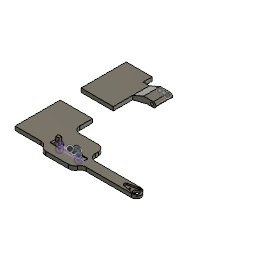
Arm (Autodesk Fusion 360 design; units mm, degrees)
part number: 2026-03-16-20-26-23-192
Autodesk Fusion 360 part; units mm, degrees
sketch "Sketch1" plane through (0, 0, 0) normal (0, 0, 1) x (1, 0, 0)
  circle A0 centre (0, 0) radius 2.9
  circle A1 centre (0, 0) radius 7.5
  line L0 (0, 0) -> (0, 7.5)
  line L1 (0, 0) -> (0, -7.5)
  line L2 (0, 7.5) -> (-100, 7.5)
  line L3 (0, -7.5) -> (-71, -7.5)
  line L4 (-100, -32.5) -> (-100, 7.5)
  line L5 (-100, 7.5) -> (-180, 7.5)
  line L6 (-180, 7.5) -> (-180, -32.5)
  line L7 (-120, -32.5) -> (-100, -32.5)
  line L8 (-100, -32.5) -> (-100, -26.5)
  line L9 (-180, 7.5) -> (-130, 7.5)
  line L10 (-130, -42.5) -> (-130, -62.5)
  line L11 (-130, -62.5) -> (-180, -62.5)
  line L12 (-180, -62.5) -> (-180, 7.5)
  arc A2 (-120, -32.5) -> (-130, -42.5) centre (-120, -42.5) ccw
  line L13 (-81, -7.5) -> (-100, -7.5)
  line L14 (-100, -7.5) -> (-100, -32.5)
  line L15 (-100, -32.5) -> (-91, -32.5)
  line L16 (-81, -22.5) -> (-81, -17.5)
  arc A3 (-71, -7.5) -> (-81, -17.5) centre (-71, -17.5) ccw
  arc A4 (-91, -32.5) -> (-81, -22.5) centre (-91, -22.5) ccw
  line L17 (-79.7998, 7.5) -> (-129.7998, 7.5)
  line L18 (-129.7998, 7.5) -> (-129.7998, 17.5)
  line L19 (-129.7998, 17.5) -> (-79.7998, 17.5)
  line L20 (-79.7998, 17.5) -> (-79.7998, 7.5)
  point P0 (-100, -7.5)
  dimension "d3" = 5.8
  dimension "d5" = 15
  dimension "d6" = 7.5
  dimension "d7" = 7.5
  dimension "d10" = 100
  dimension "d11" = 100
  dimension "d13" = 40
  dimension "d14" = 80
  dimension "d15" = 40
  dimension "d16" = 50
  dimension "d17" = 70
  dimension "d19" = 10
  dimension "d52" = 10
  dimension "d71" = 50
  dimension "d72" = 10
  constraint coincident A0.centre A1.centre
  constraint concentric A0 A1
  constraint vertical L0
  constraint parallel L0 L1
  constraint perpendicular L0 L2
  constraint perpendicular L1 L3
  constraint vertical L4
  constraint horizontal L5
  constraint vertical L6
  constraint horizontal L7
  constraint vertical L8
  constraint horizontal L9
  constraint vertical L10
  constraint horizontal L11
  constraint vertical L12
  constraint coincident L2.end L8
  constraint coincident P0 L3
  constraint coincident L6.end L7
  constraint coincident L9.end L10
  constraint tangent L7 A2
  constraint tangent L10 A2
  constraint horizontal L13
  constraint vertical L14
  constraint horizontal L15
  constraint vertical L16
  constraint coincident L13.start L16
  constraint coincident L3 L13.start
  constraint tangent L16 A3
  constraint tangent L3 A3
  constraint tangent L15 A4
  constraint tangent L16 A4
  constraint equal A3 A4
  constraint horizontal L17
  constraint vertical L18
  constraint horizontal L19
  constraint vertical L20
  constraint coincident L2 L17.start
  measures "d3" diameter of A0
  measures "d5" diameter of A1
  measures "d6" distance of A0.centre L0.end
  measures "d7" distance of A0.centre L1.end
  measures "d10" distance of L0.end L2.end
  measures "d11" distance of L1.end P0
  measures "d13" distance of L2.end L4.start
  measures "d14" distance of L2.end L5.end
  measures "d15" distance of L2.end L4.start
  measures "d16" distance of L5.end L9.end
  measures "d17" distance of L5.end L11.end
  measures "d19" radius of A2
  measures "d52" radius of A3
  measures "d71" distance of L17.start L17.end
  measures "d72" distance of L17.start L19.end
extrude "Extrude1" add sketch "Sketch1" along normal blind 6 contours A0 A1 L0 L1 | A0 A1 L0 L1 | A1 L2 L3 L4 L8 L14 L15 L16 A3 A4 L17 | L2 L5 L17 L18 L19 L20 | L4 L5 L6 L7 L8 L9 L10 L11 L12 A2 L14 L17 makes body 1
move_body "Move1" bodies 1 to x (1, 0, 0) y (0, 0, 1) z (0, -1, 0) at (0, -14.492, 14.492)
move_body "Move2" bodies 1 to x (1, 0, 0) y (0, 1, 0) z (0, 0, 1) at (0, 21, 0)
sketch "Sketch2" plane through (0, 6.508, 0) normal (0, 1, 0) x (-1, 0, 0)
  line L0 (91, -18.008) -> (120, -18.008)
  arc A0 (130, -28.008) -> (120, -18.008) centre (120, -28.008) ccw
  line L1 (130, -28.008) -> (130, -48.008)
  line L2 (130, -48.008) -> (180, -48.008)
  line L3 (180, -48.008) -> (180, 21.992)
  line L4 (180, 21.992) -> (129.7998, 21.992)
  arc A1 (0, 21.992) -> (0, 6.992) centre (0, 14.492) ccw
  line L5 (0, 6.992) -> (71, 6.992)
  line L6 (89, 17) -> (94, 17)
  line L7 (94, 17) -> (94, 13)
  line L8 (94, 13) -> (89, 13)
  line L9 (89, 13) -> (89, 17)
  arc A2 (81, -3.008) -> (71, 6.992) centre (71, -3.008) ccw
  line L10 (81, -3.008) -> (81, -8.008)
  arc A3 (81, -8.008) -> (91, -18.008) centre (91, -8.008) ccw
  line L11 (129.7998, 21.992) -> (129.7998, 31.992)
  line L12 (129.7998, 31.992) -> (79.7998, 31.992)
  line L13 (79.7998, 31.992) -> (79.7998, 21.992)
  line L14 (79.7998, 21.992) -> (0, 21.992)
  circle A4 centre (0, 14.492) radius 2.9
  dimension "d22" = 5
  dimension "d23" = 4
  constraint horizontal L6
  constraint vertical L7
  constraint horizontal L8
  constraint vertical L9
  measures "d22" distance of L6.start L6.end
  measures "d23" distance of L6.start L8.end
extrude "Extrude2" add sketch "Sketch2" along normal blind 13 contours L6 L7 L8 L9 bodies 1
sketch "Sketch3" plane through (0, 0, 13) normal (0, 0, -1) x (-1, 0, 0)
  line L0 (94, 6.508) -> (94, 19.508)
  line L1 (94, 19.508) -> (89, 19.508)
  line L2 (89, 19.508) -> (89, 6.508)
  line L3 (92.4, 13.058) -> (91.45, 13.058)
  circle A0 centre (91.45, 13.058) radius 0.95
  line L4 (120, 6.508) -> (91, 6.508)
  line L5 (91, 0.508) -> (120, 0.508)
  line L6 (120, 0.508) -> (120, 6.508)
  line L7 (91.45, 13.058) -> (91.45, 6.508)
  line L8 (91.45, 13.058) -> (94, 13.058)
  line L9 (91, 6.508) -> (91, 0.508)
  line L10 (89, 6.508) -> (94, 6.508)
  dimension "d33" = 0.95
  constraint coincident L3.end A0.centre
  constraint coincident L3.start A0
  constraint coincident L4 L7.end
  constraint perpendicular L4 L7
  constraint coincident L0 L8.end
  constraint perpendicular L0 L8
  measures "d33" distance of L3.start L3.end
extrude "Extrude3" cut sketch "Sketch3" against normal blind 10 contours L3 A0 L7 L8 | L3 A0 L7 L8 bodies 1
sketch "Sketch4" plane through (0, 6.508, 0) normal (0, 1, 0) x (-1, 0, 0)
  line L0 (94, 17) -> (94, 13)
  line L1 (91, -18.008) -> (120, -18.008)
  arc A0 (130, -28.008) -> (120, -18.008) centre (120, -28.008) ccw
  line L2 (130, -28.008) -> (130, -48.008)
  line L3 (130, -48.008) -> (180, -48.008)
  line L4 (180, -48.008) -> (180, 21.992)
  line L5 (180, 21.992) -> (129.7998, 21.992)
  arc A1 (0, 21.992) -> (0, 6.992) centre (0, 14.492) ccw
  line L6 (0, 6.992) -> (71, 6.992)
  line L7 (94, 17) -> (116.7, 17)
  arc A2 (81, -3.008) -> (71, 6.992) centre (71, -3.008) ccw
  line L8 (81, -3.008) -> (81, -8.008)
  arc A3 (81, -8.008) -> (91, -18.008) centre (91, -8.008) ccw
  line L9 (116.7, 17) -> (116.8, 17)
  line L10 (116.8, 17) -> (121.8, 17)
  line L11 (121.8, 17) -> (121.8, 13)
  line L12 (121.8, 13) -> (116.8, 13)
  line L13 (116.8, 13) -> (116.8, 17)
  line L14 (89, 13) -> (89, 17)
  line L15 (89, 17) -> (94, 17)
  line L16 (94, 13) -> (89, 13)
  line L17 (129.7998, 21.992) -> (129.7998, 31.992)
  line L18 (129.7998, 31.992) -> (79.7998, 31.992)
  line L19 (79.7998, 31.992) -> (79.7998, 21.992)
  line L20 (79.7998, 21.992) -> (0, 21.992)
  circle A4 centre (0, 14.492) radius 2.9
  dimension "d38" = 22.7
  dimension "d53" = 0.1
  dimension "d54" = 5
  dimension "d55" = 4
  constraint coincident L0 L7.start
  constraint perpendicular L0 L7
  constraint horizontal L9
  constraint horizontal L10
  constraint vertical L11
  constraint horizontal L12
  constraint vertical L13
  measures "d38" distance of L0.start L7.end
  measures "d53" distance of L7.end L9.end
  measures "d54" distance of L9.end L10.end
  measures "d55" distance of L9.end L12.end
extrude "Extrude4" add sketch "Sketch4" along normal blind 13 contours L10 L11 L12 L13 bodies 1
sketch "Sketch6" plane through (0, 0, 13) normal (0, 0, -1) x (-1, 0, 0)
  line L0 (121.8, 6.508) -> (121.8, 19.508)
  line L1 (121.8, 19.508) -> (116.8, 19.508)
  line L2 (116.8, 19.508) -> (116.8, 6.508)
  line L3 (122.7377, 11.508) -> (116.8, 11.508)
  line L4 (116.8, 11.508) -> (116.8, 6.508)
  line L5 (116.8, 6.508) -> (130.8, 6.508)
  spline S0 degree 3 poles (122.7377, 11.508) (123.0614, 10.8558) (123.4874, 10.2087) (124.46, 9.0768) (125.006, 8.5907) (126.304, 7.6534) (127.188, 7.2097) (129.0062, 6.6373) (129.9408, 6.508) (130.8, 6.508) knots 2.617897 2.617897 2.617897 2.617897 2.836337 2.836337 3.054776 3.054776 3.376245 3.376245 3.697714 3.697714 3.697714 3.697714
  line L6 (120, 6.508) -> (130, 6.508)
  line L7 (120, 6.508) -> (120, 0.508)
  line L8 (130, 0.508) -> (120, 0.508)
  line L9 (130, 0.508) -> (130, 6.508)
  line L10 (120, 6.508) -> (91, 6.508)
  line L11 (91, 6.508) -> (91, 0.508)
  line L12 (91, 0.508) -> (120, 0.508)
  line L13 (120, 0.508) -> (120, 6.508)
  line L14 (116.8, 6.508) -> (119.35, 6.508)
  line L15 (119.35, 6.508) -> (119.35, 13.058)
  line L16 (119.35, 13.058) -> (116.8, 13.058)
  line L17 (116.8, 13.058) -> (116.8, 6.508)
  circle A0 centre (119.35, 13.058) radius 0.95
  line L18 (116.8, 6.508) -> (121.8, 6.508)
  dimension "d73" = 2.55
  dimension "d74" = 6.55
  dimension "d75" = 1.9
  constraint horizontal L14
  constraint vertical L15
  constraint horizontal L16
  constraint vertical L17
  constraint coincident L2.end L4.end
  constraint coincident L15.end L16.start
  measures "d73" distance of L2.end L14.end
  measures "d74" distance of L2.end L16.end
  measures "d75" diameter of A0
extrude "Extrude7" cut sketch "Sketch6" against normal blind 10 contours L15 L16 A0 | L15 L16 A0 bodies 1
fillet "Fillet11" radius 10 2 edges at (-129.7998, 3.508, 21.992) (-79.7998, 3.508, 21.992) on bodies 1
fillet "Fillet12" radius 10 2 edges at (-129.7998, 3.508, 31.992) (-79.7998, 3.508, 31.992) on bodies 1
fillet "Fillet13" radius 9 2 edges at (-121.8, 6.508, 15) (-89, 6.508, 15) on bodies 1
sketch "Sketch7" plane through (0, 6.508, 0) normal (0, 1, 0) x (-1, 0, 0)
  line L0 (94, 17) -> (94, 13)
  line L1 (94, 13) -> (80, 13)
  line L2 (80, 13) -> (80, 17)
  line L3 (130.8, 13) -> (116.8, 13)
  line L4 (116.8, 13) -> (116.8, 17)
  line L5 (130.8, 17) -> (130.8, 13)
  arc A0 (87.1203, 31.992) -> (78.4601, 26.992) centre (87.1203, 21.992) ccw
  arc A1 (69.7998, 21.992) -> (78.4601, 26.992) centre (69.7998, 31.992) ccw
  line L6 (69.7998, 21.992) -> (0, 21.992)
  arc A2 (0, 21.992) -> (0, 6.992) centre (0, 14.492) ccw
  line L7 (0, 6.992) -> (71, 6.992)
  arc A3 (81, -3.008) -> (71, 6.992) centre (71, -3.008) ccw
  line L8 (81, -3.008) -> (81, -8.008)
  arc A4 (81, -8.008) -> (91, -18.008) centre (91, -8.008) ccw
  line L9 (91, -18.008) -> (120, -18.008)
  arc A5 (130, -28.008) -> (120, -18.008) centre (120, -28.008) ccw
  line L10 (130, -28.008) -> (130, -48.008)
  line L11 (130, -48.008) -> (180, -48.008)
  line L12 (180, -48.008) -> (180, 21.992)
  line L13 (180, 21.992) -> (139.7998, 21.992)
  arc A6 (131.1396, 26.992) -> (139.7998, 21.992) centre (139.7998, 31.992) ccw
  arc A7 (131.1396, 26.992) -> (122.4793, 31.992) centre (122.4793, 21.992) ccw
  line L14 (122.4793, 31.992) -> (87.1203, 31.992)
  line L15 (94, 13) -> (94, 8)
  line L16 (94, 8) -> (81, 8)
  line L17 (81, 8) -> (81, -3.008)
  line L18 (94, -3.008) -> (94, 8)
  line L19 (81, 8) -> (180, 8)
  line L20 (180, 8) -> (180, -18.008)
  line L21 (120, -18.008) -> (91, -18.008)
  line L22 (81, -8.008) -> (81, 8)
  line L23 (130, -48.008) -> (180, -48.008)
  line L24 (180, -48.008) -> (180, -18.008)
  line L25 (180, -18.008) -> (130, -18.008)
  line L26 (130, -28.008) -> (130, -48.008)
  arc A8 (81, -8.008) -> (91, -18.008) centre (91, -8.008) ccw
  arc A9 (130, -28.008) -> (120, -18.008) centre (120, -28.008) ccw
  line L27 (180, 8) -> (139.7998, 8)
  line L28 (139.7998, 8) -> (139.7998, 21.992)
  line L29 (139.7998, 21.992) -> (180, 21.992)
  line L30 (180, 21.992) -> (180, 8)
  line L31 (130, -28.008) -> (130, 8)
  circle A10 centre (0, 14.492) radius 2.9
  line L32 (80, 17) -> (94, 17)
  line L33 (116.8, 17) -> (130.8, 17)
  dimension "d84" = 5
  constraint coincident L0.end L1.start
  constraint perpendicular L1 L15
  constraint horizontal L16
  constraint vertical L17
  constraint vertical L18
  constraint coincident A3.start L8.start
  constraint horizontal L19
  constraint vertical L20
  constraint horizontal L21
  constraint vertical L22
  constraint coincident L12 L20.end
  constraint horizontal L23
  constraint vertical L24
  constraint horizontal L25
  constraint vertical L26
  constraint coincident L10.end L11.start
  constraint tangent L21 A8
  constraint tangent L22 A8
  constraint coincident L20.end L21
  constraint coincident L25.end L26
  constraint tangent L21 A9
  constraint tangent L26 A9
  constraint equal A8 A9
  constraint horizontal L27
  constraint vertical L28
  constraint horizontal L29
  constraint vertical L30
  constraint coincident L13.end A6.end
  constraint coincident A5.start L10.start
  constraint coincident L19 L31.end
  constraint tangent A5 L31
  measures "d84" distance of L0.end L15.end
extrude "Extrude8" add sketch "Sketch7" along normal blind 6 from surface at 10 separate body contours L12 L13 L19 L27 L28 L29 L30 | L12 L19 L20 L25 L27 L31 | L10 L11 L12 L23 L24 L25 L26 L31 makes body 2
sketch "Sketch8" plane through (0, 0, 17) normal (0, 0, 1) x (1, 0, 0)
  arc A0 (-89, 15.508) -> (-80, 6.508) centre (-80, 15.508) ccw
  line L0 (-89, 15.508) -> (-89, 19.508)
  line L1 (-89, 19.508) -> (-94, 19.508)
  line L2 (-94, 19.508) -> (-94, 6.508)
  circle A1 centre (-91.45, 13.058) radius 0.95
  line L3 (-94, 13) -> (-100, 13)
  circle A2 centre (-100, 13) radius 1.8
  line L4 (-94, 6.508) -> (-80, 6.508)
  dimension "d91" = 6
  dimension "d92" = 3.6
  constraint coincident L2 L3.start
  constraint perpendicular L2 L3
  constraint coincident L3.end A2.centre
  measures "d91" distance of L3.start L3.end
  measures "d92" diameter of A2
sketch "Sketch9" plane through (0, 0, 8) normal (0, 0, 1) x (1, 0, 0)
  line L0 (-139.7998, 16.508) -> (-130, 16.508)
  line L1 (-130, 16.508) -> (-130, 22.508)
  line L2 (-130, 22.508) -> (-139.7998, 22.508)
  line L3 (-139.7998, 22.508) -> (-139.7998, 16.508)
  line L4 (-94, 10) -> (-107, 10)
  line L5 (-107, 10) -> (-107, 15)
  line L6 (-94, 15) -> (-94, 10)
  circle A0 centre (-100, 13) radius 1.8
  line L7 (-94, 10) -> (-107, 10)
  line L8 (-107, 10) -> (-107, 16)
  line L9 (-107, 16) -> (-94, 16)
  line L10 (-94, 16) -> (-94, 10)
  line L11 (-94, 17) -> (-108, 17)
  line L12 (-108, 17) -> (-108, 9)
  line L13 (-108, 9) -> (-94, 9)
  line L14 (-94, 9) -> (-94, 17)
  line L15 (-108, 17) -> (-130, 22.508)
  line L16 (-108, 9) -> (-113, 9)
  line L17 (-113, 9) -> (-130, 16.508)
  dimension "d93" = 13
  dimension "d94" = 6
  constraint horizontal L4
  constraint vertical L5
  constraint vertical L6
  constraint horizontal L7
  constraint vertical L8
  constraint horizontal L9
  constraint vertical L10
  constraint horizontal L11
  constraint vertical L12
  constraint horizontal L13
  constraint vertical L14
  constraint coincident L1.end L2.start
  constraint coincident L0.end L1.start
  constraint perpendicular L12 L16
  measures "d93" distance of L4.start L4.end
  measures "d94" distance of L4.start L9.end
extrude "Extrude9" add sketch "Sketch9" against normal blind 26 contours L1 L12 L15 L16 L17 | L4 L5 L7 L8 L9 L11 L12 L13 L14 | L4 L5 L6 L7 L8 L9 L10 L14 bodies 2
extrude "Extrude10" add sketch "Sketch9" against normal blind 20 from surface at -6 contours A0 bodies 2
move_body "Move3" bodies 2 to x (1, 0, 0) y (0, -1, 0) z (0, 0, -1) at (0, 20, -96.0161)
move_body "Move4" bodies 2 to x (1, 0, 0) y (0, 1, 0) z (0, 0, 1) at (0, 2.508, -31.992)
move_body "Move5" bodies 1 to x (1, 0, 0) y (0, 1, 0) z (0, 0, 1) at (0, -0.508, 0)
sketch "Sketch12" plane through (0, 0, -136.008) normal (0, 0, -1) x (-1, 0, 0)
  line L0 (130, 0) -> (139.7998, 0)
  line L1 (139.7998, 0) -> (139.7998, 6)
  line L2 (139.7998, 6) -> (130, 6)
  circle A0 centre (100, 9.508) radius 3.5
  line L3 (100, 9.508) -> (116, 9.508)
  circle A1 centre (116, 9.508) radius 2
  circle A2 centre (100, 9.508) radius 1.8
  line L4 (130, 6) -> (113, 13.508)
  line L5 (113, 13.508) -> (94, 13.508)
  line L6 (94, 13.508) -> (94, 5.508)
  line L7 (94, 5.508) -> (108, 5.508)
  line L8 (108, 5.508) -> (130, 0)
  line L9 (100.3281, 12.9926) -> (116.1875, 11.4992)
  line L10 (116.1875, 7.5169) -> (100.3281, 6.0235)
  dimension "d125" = 7
  dimension "d126" = 16
  dimension "d127" = 4
  constraint coincident A0.centre L3.start
  constraint horizontal L3
  constraint coincident L3.end A1.centre
  constraint coincident A0 L9.start
  constraint coincident A1 L9.end
  constraint coincident A1 L10.start
  constraint coincident A0 L10.end
  constraint tangent A0 L9
  constraint tangent A0 L10
  constraint tangent A1 L10
  constraint tangent A1 L9
  measures "d125" diameter of A0
  measures "d126" distance of A0.centre L3.end
  measures "d127" diameter of A1
fillet "Fillet17" radius 4 2 edges at (-94, 13.508, -123.008) (-94, 5.508, -123.008) on bodies 2
extrude "Extrude12" cut sketch "Sketch12" against normal blind 2 contours A0 | A0 L3 A1 L10 | A0 L3 A1 L9 | A1 bodies 2
sketch "Sketch13" plane through (0, 0, -134.008) normal (0, 0, -1) x (-1, 0, 0)
  circle A0 centre (100, 9.508) radius 1.8
  arc A1 (100.3281, 12.9926) -> (100.3281, 6.0235) centre (100, 9.508) ccw
  line L0 (100.3281, 6.0235) -> (116.1875, 7.5169)
  arc A2 (116.1875, 7.5169) -> (116.1875, 11.4992) centre (116, 9.508) ccw
  line L1 (116.1875, 11.4992) -> (100.3281, 12.9926)
  line L2 (100, 9.508) -> (106, 9.508)
  circle A3 centre (106, 9.508) radius 0.5
  line L3 (106, 9.508) -> (112, 9.508)
  circle A4 centre (112, 9.508) radius 0.5
  circle A5 centre (100, 9.508) radius 2.2
  dimension "d132" = 6
  dimension "d133" = 1
  dimension "d136" = 6
  dimension "d137" = 1
  dimension "d138" = 4.4
  constraint coincident A0.centre A1.centre
  constraint horizontal L2
  constraint coincident L2.end A3.centre
  constraint parallel L2 L3
  constraint coincident L3.end A4.centre
  measures "d132" distance of A0.centre L2.end
  measures "d133" diameter of A3
  measures "d136" distance of L2.end L3.end
  measures "d137" diameter of A4
  measures "d138" diameter of A5
extrude "Extrude13" cut sketch "Sketch13" against normal blind 5 contours L2 A3 L3 | L2 A3 L3 | A4 bodies 2
sketch "Sketch14" plane through (0, 0, -130.008) normal (0, 0, -1) x (-1, 0, 0)
  circle A0 centre (100, 9.508) radius 1.8
extrude "Extrude14" cut sketch "Sketch13" against normal blind 50 contours A0 | A5 bodies 2
sketch "Sketch15" plane through (0, 6, 0) normal (0, 1, 0) x (-1, 0, 0)
  line L0 (94, 17) -> (94, 13)
  line L1 (94, 13) -> (80, 13)
  line L2 (80, 13) -> (80, 17)
  line L3 (130.8, 13) -> (116.8, 13)
  line L4 (116.8, 13) -> (116.8, 17)
  line L5 (130.8, 17) -> (130.8, 13)
  circle A0 centre (0, 14.492) radius 2.9
  arc A1 (87.1203, 31.992) -> (78.4601, 26.992) centre (87.1203, 21.992) ccw
  arc A2 (69.7998, 21.992) -> (78.4601, 26.992) centre (69.7998, 31.992) ccw
  line L6 (69.7998, 21.992) -> (0, 21.992)
  arc A3 (0, 21.992) -> (0, 6.992) centre (0, 14.492) ccw
  line L7 (0, 6.992) -> (71, 6.992)
  arc A4 (81, -3.008) -> (71, 6.992) centre (71, -3.008) ccw
  line L8 (81, -3.008) -> (81, -8.008)
  arc A5 (81, -8.008) -> (91, -18.008) centre (91, -8.008) ccw
  line L9 (91, -18.008) -> (120, -18.008)
  arc A6 (130, -28.008) -> (120, -18.008) centre (120, -28.008) ccw
  line L10 (130, -28.008) -> (130, -48.008)
  line L11 (130, -48.008) -> (180, -48.008)
  line L12 (180, -48.008) -> (180, 21.992)
  line L13 (180, 21.992) -> (139.7998, 21.992)
  arc A7 (131.1396, 26.992) -> (139.7998, 21.992) centre (139.7998, 31.992) ccw
  arc A8 (131.1396, 26.992) -> (122.4793, 31.992) centre (122.4793, 21.992) ccw
  line L14 (122.4793, 31.992) -> (87.1203, 31.992)
  circle A9 centre (0, 14.492) radius 4.4
  circle A10 centre (0, 14.492) radius 6
  line L15 (0, 14.492) -> (16, 14.492)
  circle A11 centre (16, 14.492) radius 2.75
  line L16 (1.2187, 20.3669) -> (16.5586, 17.1847)
  line L17 (16.5586, 11.7993) -> (1.2188, 8.6171)
  line L18 (0, 14.492) -> (10, 14.492)
  circle A12 centre (10, 14.492) radius 1.15
  line L19 (0, 14.492) -> (0, 8.492)
  line L20 (0, 14.492) -> (0, 20.492)
  circle A13 centre (-10, 14.492) radius 1.15
  circle A14 centre (-16, 14.492) radius 2.75
  line L21 (-16.5586, 11.7993) -> (-1.2188, 8.6171)
  line L22 (0, 14.492) -> (-16, 14.492)
  line L23 (-1.2187, 20.3669) -> (-16.5586, 17.1847)
  line L24 (20.9721, 21.992) -> (20.3038, 21.992)
  line L25 (80, 17) -> (94, 17)
  line L26 (116.8, 17) -> (130.8, 17)
  point P0 (-10, 14.492)
  dimension "d141" = 8.8
  dimension "d144" = 12
  dimension "d145" = 16
  dimension "d146" = 5.5
  dimension "d149" = 10
  dimension "d150" = 2.3
  constraint horizontal L15
  constraint coincident A0.centre A3.centre
  constraint coincident L15.end A11.centre
  constraint coincident A10 L16.start
  constraint coincident A11 L16.end
  constraint coincident A11 L17.start
  constraint coincident A10 L17.end
  constraint tangent A10 L16
  constraint tangent A11 L16
  constraint tangent A11 L17
  constraint tangent A10 L17
  constraint parallel L15 L18
  constraint coincident L18.end A12.centre
  constraint coincident A10 L19.end
  constraint perpendicular L15 L19
  constraint coincident A10 L20.end
  constraint perpendicular L18 L20
  constraint coincident L6 L24.start
  constraint coincident L6 L24.end
  measures "d141" diameter of A9
  measures "d144" diameter of A10
  measures "d145" distance of A0.centre L15.end
  measures "d146" diameter of A11
  measures "d149" distance of A0.centre L18.end
  measures "d150" diameter of A12
extrude "Extrude15" cut sketch "Sketch15" against normal blind 10 contours A0 A9 L15 L18 L19 | A0 A9 L15 L18 L20 | A0 A9 L20 L22 | A0 A9 L19 L22 bodies 1
extrude "Extrude16" cut sketch "Sketch15" against normal blind 2.4 contours A9 A10 L15 L18 L19 | A9 A10 L15 L18 L20 | A9 A10 L20 L22 | A9 A10 L19 L22 | A10 L15 A11 L17 L18 A12 | A10 L15 A11 L16 L18 A12 | L15 L18 A12 | L15 L18 A12 | A11 bodies 1
extrude "Extrude17" cut sketch "Sketch15" against normal blind 10 contours L15 L18 A12 | L15 L18 A12 bodies 1
extrude "Extrude18" cut sketch "Sketch15" against normal blind 2.4 contours A3 A10 L22 L23 | A3 A10 L21 L22 bodies 1
fillet "Fillet18" radius 4 2 edges at (-123.8, 6, 13) (-87, 6, 13) on bodies 1
